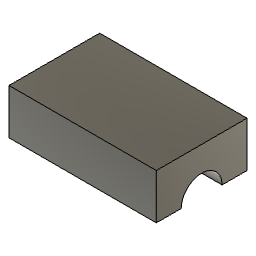
box2 (Autodesk Fusion 360 design; units mm, degrees)
Autodesk Fusion 360 part; units mm, degrees
sketch "Sketch1" plane through (0, 0, 0) normal (1, 0, 0) x (0, 1, 0)
  line L0 (-20, -10) -> (20, -10)
  line L1 (20, -10) -> (20, 10)
  line L2 (20, 10) -> (-20, 10)
  line L3 (-20, 10) -> (-20, -10)
  dimension "d1" = 20
  dimension "d2" = 40
  dimension "d3" = 20
  dimension "d4" = 10
  constraint horizontal L0
  constraint vertical L1
  constraint horizontal L2
  constraint vertical L3
  measures "d1" distance of L0.start L2.end
  measures "d2" distance of L1.end L2.end
  measures "d3" distance of origin L3
  measures "d4" distance of origin L2
extrude "Extrude1" add sketch "Sketch1" along normal blind 65
sketch "Sketch2" plane through (65, 0, 0) normal (1, 0, 0) x (0, 1, 0)
  line L0 (-20, 10) -> (-20, -10)
  line L1 (-20, -10) -> (20, -10)
  line L2 (20, -10) -> (20, 10)
  line L3 (20, 10) -> (-20, 10)
  circle A0 centre (0, -10) radius 9
  dimension "d7" = 18
  constraint midpoint L1 A0.centre
  measures "d7" diameter of A0
extrude "Extrude2" cut sketch "Sketch2" against normal blind 55 contours L1 A0 picked at (-1.096, -7.2074)
sketch "Sketch3" plane through (65, 0, 0) normal (1, 0, 0) x (0, 1, 0)
  arc A0 (9, -10) -> (-9, -10) centre (0, -10) ccw
  line L0 (9, -10) -> (20, -10)
  line L1 (20, -10) -> (20, 10)
  line L2 (20, 10) -> (-20, 10)
  line L3 (-20, 10) -> (-20, -10)
  line L4 (-20, -10) -> (-9, -10)
  circle A1 centre (0, -10) radius 17
  dimension "d10" = 34
  constraint concentric A0 A1
  measures "d10" diameter of A1
extrude "Extrude3" cut sketch "Sketch3" against normal blind 6 from surface at -9 contours A0 L0 L4 A1 picked at (-13.3871, -4.9868)
extrude "Extrude4" cut sketch "Sketch3" against normal blind 6 from surface at -19 contours A0 L0 L4 A1 picked at (-13.3871, -4.9868)
extrude "Extrude5" cut 1 faces at (40, -13.3871, -4.9868) along direction (-1, 0, 0) blind 6 from surface at 4
extrude "Extrude6" cut 1 faces at (30, -13.3871, -4.9868) along direction (-1, 0, 0) blind 6 from surface at 4
extrude "Extrude7" cut 1 faces at (20, -13.3871, -4.9868) along direction (-1, 0, 0) blind 6 from surface at 4
sketch "Sketch5" plane through (10, 0, 0) normal (1, 0, 0) x (0, 1, 0)
  line L0 (-17, -10) -> (17, -10)
  arc A0 (17, -10) -> (-17, -10) centre (0, -10) ccw
  circle A1 centre (0, -10) radius 2
  dimension "d26" = 4
  constraint concentric A0 A1
  measures "d26" diameter of A1
extrude "Extrude8" cut sketch "Sketch5" against normal blind 5 contours L0 A1 picked at (0.4157, -9.4788)
